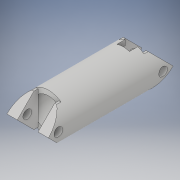
# Autodesk Inventor part: Middle Finger Summ
Saved by Autodesk Inventor 2017 (Build 210142000, 142)
## iProperties
Created: 2018-11-19
Part Number: Middle Finger Summ
Material: Generic
Document SubType Name: Modeling
Designer: S346795925
Density: 1 g/cm^3
Appearance: Default
Author: S346795925
Autodesk Inventor part; units mm, degrees
ref_plane "XZ Plane" through (0, 0, 0) normal (0, 1, 0) x (-1, 0, 0)
sketch "Sketch1" plane through (0, 0, 0) normal (0, 0, 1) x (1, 0, 0)
  circle A0 centre (0, 0) radius 6.35
  circle A1 centre (0, 0) radius 4.826
  dimension "d0" = 12.7
  dimension "d23" = 1.524
  constraints: 2 centre point, 2 coincident
  measures "d0" diameter of A0
  measures "d23" radial gap between concentric circles of A1 A0
extrude "Extrusion1" add sketch "Sketch1" along normal blind 25.4
ref_plane "Work Plane1" through (-3.175, 0, 0) normal (1, 0, 0) x (0, 1, 0)
sketch "Sketch2" plane through (-3.175, 0, 0) normal (1, 0, 0) x (0, 1, 0)
  line L0 (0, 0) -> (5.08, 0)
  line L1 (-6.35, 0) -> (6.35, 0) projected
  line L2 (5.08, 0) -> (5.08, -1.27)
  line L3 (0, -6.35) -> (0, -6.35)
  line L4 (-5.08, -1.27) -> (-5.08, 0)
  line L5 (-5.08, 0) -> (0, 0)
  line L6 (5.08, -1.27) -> (0, -6.35)
  line L7 (0, -6.35) -> (-5.08, -1.27)
  circle A0 centre (0, -3.302) radius 1.3208
  point P0 (5.08, -6.35)
  point P1 (-5.08, -6.35)
  dimension "d5" = 5.08
  dimension "d6" = 6.35
  dimension "d7" = 90
  dimension "d8" = 10.16
  dimension "d9" = 90
  dimension "d10" = 5.08
  dimension "d11" = 5.08
  dimension "d12" = 5.08
  dimension "d13" = 5.08
  dimension "d14" = 2.6416
  dimension "d15" = 3.302
  constraints: 14 end point, 6 point on line, 4 perpendicular, 1 centre point
  measures "d5" distance of L0.start L0.end
  measures "d6" distance of L0.end point (5.08, -6.35)
  measures "d7" angle of L0 L2
  measures "d8" distance of point (5.08, -6.35) point (-5.08, -6.35)
  measures "d9" angle of L2 L3
  measures "d10" distance of L2.end point (5.08, -6.35)
  measures "d11" distance of L3.start point (5.08, -6.35)
  measures "d12" distance of L3.end point (-5.08, -6.35)
  measures "d13" distance of L4.start point (-5.08, -6.35)
  measures "d14" diameter of A0
  measures "d15" distance from line of L1 A0.centre
extrude "Extrusion2" add sketch "Sketch2" against normal up to surface round surface about axis through (0, 0, 0) along (0, 0, 1) radius 6.35 far side no
mirror "Mirror1" about plane through (0, 0, 0) normal (1, 0, 0) of "Extrusion2"
ref_plane "Work Plane2" through (0, 0, 12.7) normal (0, 0, 1) x (1, 0, 0)
mirror "Mirror2" about plane through (0, 0, 12.7) normal (0, 0, 1) of "Extrusion2", "Mirror1"
sketch "Sketch3" plane through (0, 0, 0) normal (0, 1, 0) x (-1, 0, 0)
  line L0 (-1.905, -2.54) -> (1.905, -2.54)
  line L1 (1.905, -2.54) -> (1.905, 2.54)
  line L2 (1.905, 2.54) -> (-1.905, 2.54)
  line L3 (-1.905, 2.54) -> (-1.905, -2.54)
  line L4 (-1.905, -2.54) -> (1.905, 2.54) construction
  line L5 (1.905, -2.54) -> (-1.905, 2.54) construction
  point P0 (0, 0)
  dimension "d19" = 3.81
  dimension "d20" = 5.08
  constraints: 12 end point, 2 midpoint, 2 parallel, 1 horizontal, 1 perpendicular
  measures "d19" distance of L2.end L1.end
  measures "d20" distance of L1.end L0.end
extrude "Extrusion3" cut sketch "Sketch3" along normal up to surface round surface about axis through (0, 0, 0) along (0, 0, 1) radius 6.35 far side no
equation "\"d11\" = d10"
equation "\"d12\" = d10"
equation "\"d13\" = d12"
body "Solid1"
